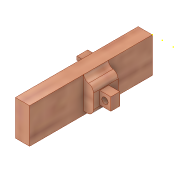
# Autodesk Inventor part: pen holder
Saved by Autodesk Inventor 2019 (Build 230136000, 136)
## iProperties
Created: 2020-02-13
Part Number: pen holder
Material: Wood (Oak)
Document SubType Name: Modeling
Designer: Admin
Density: 0.76 g/cm^3
Appearance: White Oak - Natural Medium Gloss
Author: Admin
Autodesk Inventor part; units mm, degrees
ref_plane "YZ Plane" through (0, 0, 0) normal (1, 0, 0) x (0, 1, 0)
ref_plane "XZ Plane" through (0, 0, 0) normal (0, 1, 0) x (-1, 0, 0)
ref_plane "XY Plane" through (0, 0, 0) normal (0, 0, 1) x (1, 0, 0)
sketch "Sketch1" plane through (0, 0, 0) normal (0, 0, 1) x (1, 0, 0)
  line L0 (0, 0) -> (2.9424, 0)
  line L1 (2.9424, 0) -> (2.9424, -7.2806)
  line L2 (2.9424, -7.2806) -> (0, -7.2806)
  line L3 (0, -7.2806) -> (0, 0)
  constraints: 8 end point, 2 parallel, 1 horizontal, 1 perpendicular
extrude "Extrusion1" add sketch "Sketch1" along normal blind 25.4
sketch "Sketch2" plane through (2.9424, -7.2806, 0) normal (1, 0, 0) x (0, 0, -1)
  point P0 (0, 7.2806)
sketch "Sketch3" plane through (2.9424, -7.2806, 0) normal (1, 0, 0) x (0, 0, -1)
  line L0 (-9.1297, 6.2288) -> (-14.2174, 6.2288)
  line L1 (-14.2174, 6.2288) -> (-14.2174, 0.7246)
  line L2 (-14.2174, 0.7246) -> (-9.1297, 0.7246)
  line L3 (-9.1297, 0.7246) -> (-9.1297, 6.2288)
  point P0 (0, 7.2806)
  constraints: 8 end point, 2 parallel, 1 horizontal, 1 perpendicular
extrude "Extrusion2" add sketch "Sketch3" along normal blind 2.032
fillet "Fillet1" radius 1.27 3 edges at (4.9744, -1.0519, 11.6735) (4.9744, -6.556, 11.6735) (2.9424, -1.0519, 11.6735)
sketch "Sketch4" plane through (4.9744, -7.2806, 0) normal (1, 0, 0) x (0, 0, -1)
  line L0 (-12.9198, 2.186) -> (-11.0597, 2.186)
  line L1 (-11.0597, 2.186) -> (-11.0597, 4.7902)
  line L2 (-11.0597, 4.7902) -> (-12.9198, 4.7902)
  line L3 (-12.9198, 4.7902) -> (-12.9198, 2.186)
  point P0 (0, 7.2806)
  constraints: 8 end point, 2 parallel, 1 horizontal, 1 perpendicular
extrude "Extrusion3" add sketch "Sketch4" along normal blind 2.286
sketch "Sketch5" plane through (4.9744, -7.2806, 0) normal (1, 0, 0) x (0, 0, -1)
  point P0 (0, 7.2806)
sketch "Sketch6" plane through (7.2604, -3.8837, 11.7408) normal (1, 0, 0) x (0, 0, -1)
  point P0 (11.7408, 3.8837)
sketch "Sketch7" plane through (4.9744, -5.0946, 12.9198) normal (0, 0, 1) x (1, 0, 0)
  circle A0 centre (1.0916, 1.297) radius 0.6417
  point P0 (-4.9744, 5.0946)
  constraints: 1 centre point
extrude "Extrusion4" cut sketch "Sketch7" against normal blind 25.4
sketch "Sketch8" plane through (0, -7.2806, 0) normal (0, -1, 0) x (1, 0, 0)
  point P0 (0, 0)
sketch "Sketch9" plane through (0, -7.2806, 0) normal (-1, 0, 0) x (0, 0, 1)
  line L0 (8.6535, 6.5442) -> (10.8988, 6.5442)
  line L1 (10.8988, 6.5442) -> (10.8988, 5.8257)
  line L2 (10.8988, 5.8257) -> (8.6535, 5.8257)
  line L3 (8.6535, 5.8257) -> (8.6535, 6.5442)
  point P0 (0, 7.2806)
  constraints: 8 end point, 2 parallel, 1 horizontal, 1 perpendicular
extrude "Extrusion5" add sketch "Sketch9" along normal blind 1.778
sketch "Sketch10" plane through (0, -7.2806, 0) normal (-1, 0, 0) x (0, 0, 1)
  line L0 (9.1297, 1.9946) -> (14.2174, 1.9946) projected
  line L1 (8.5112, 2.6437) -> (10.4941, 2.6437)
  line L2 (10.4941, 2.6437) -> (10.4941, 1.9946)
  line L3 (10.4941, 1.9946) -> (8.5112, 1.9946)
  line L4 (8.5112, 1.9946) -> (8.5112, 2.6437)
  point P0 (0, 7.2806)
  constraints: 8 end point, 2 parallel, 1 horizontal, 1 perpendicular, 1 point on line
extrude "Extrusion6" add sketch "Sketch10" along normal blind 1.778
body "Solid1"
